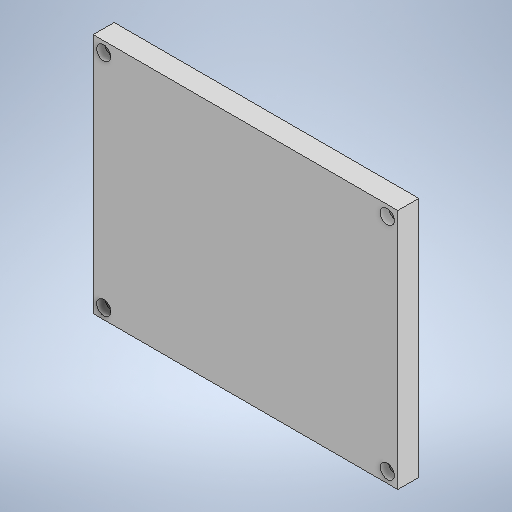
# Autodesk Inventor part: boden
Saved by Autodesk Inventor 2027 (Build 310192060, 192F)
## iProperties
Created: 2026-06-16
Part Number: boden
Material: Generic
Document SubType Name: Modeling
Designer: Felix
Density: 1 g/cm^3
Appearance: Default
Author: Felix
Autodesk Inventor part; units mm, degrees
ref_plane "YZ Plane" through (0, 0, 0) normal (1, 0, 0) x (0, 1, 0)
ref_plane "XZ Plane" through (0, 0, 0) normal (0, 1, 0) x (-1, 0, 0)
ref_plane "XY Plane" through (0, 0, 0) normal (0, 0, 1) x (1, 0, 0)
sketch "Sketch3" plane through (0, 0, 0) normal (0, 0, 1) x (1, 0, 0)
  line L0 (0, 0) -> (145, 0)
  line L1 (145, 0) -> (145, 115)
  line L2 (145, 115) -> (0, 115)
  line L3 (0, 115) -> (0, 0)
  dimension "d24" = 145
  dimension "d25" = 115
  constraints: 8 end point, 2 parallel, 1 horizontal, 1 perpendicular
  measures "d24" distance of L2.end L1.end
  measures "d25" distance of L1.end L0.end
extrude "Extrusion1" add sketch "Sketch3" along normal blind 10
sketch "Sketch1" plane through (0, 0, 0) normal (0, 0, 1) x (1, 0, 0)
  circle A0 centre (15, 43) radius 2
  circle A1 centre (62, 43) radius 2
  circle A2 centre (15, 20) radius 2
  circle A3 centre (20, 95) radius 2
  circle A4 centre (78, 95) radius 2
  circle A5 centre (20, 63) radius 2
  circle A6 centre (97, 56.9) radius 2
  circle A7 centre (133.9, 56.9) radius 2
  circle A8 centre (97, 20) radius 2
  point P0 (0, 0)
  point P1 (3.899, 77.9301)
  dimension "d0" = 4
  dimension "d1" = 4
  dimension "d2" = 4
  dimension "d3" = 23
  dimension "d4" = 47
  dimension "d6" = 4
  dimension "d7" = 4
  dimension "d8" = 4
  dimension "d9" = 32
  dimension "d10" = 58
  dimension "d11" = 5
  dimension "d12" = 20
  dimension "d13" = 4
  dimension "d14" = 4
  dimension "d15" = 4
  dimension "d16" = 36.9
  dimension "d17" = 36.9
  dimension "d18" = 35
  dimension "d28" = 20
  dimension "d29" = 15
  constraints: 9 centre point, 4 horizontal alignment, 3 vertical alignment
  measures "d0" diameter of A0
  measures "d1" diameter of A1
  measures "d2" diameter of A2
  measures "d3" distance of A2.centre A0.centre
  measures "d4" distance of A1.centre A0.centre
  measures "d6" diameter of A3
  measures "d7" diameter of A4
  measures "d8" diameter of A5
  measures "d9" distance of A5.centre A3.centre
  measures "d10" distance of A4.centre A3.centre
  measures "d11" horizontal distance of A0.centre A5.centre
  measures "d12" vertical distance of A0.centre A5.centre
  measures "d13" diameter of A6
  measures "d14" diameter of A7
  measures "d15" diameter of A8
  measures "d16" distance of A8.centre A6.centre
  measures "d17" distance of A7.centre A6.centre
  measures "d18" horizontal distance of A8.centre A1.centre
  measures "d28" vertical distance of point (0, 0) A2.centre
  measures "d29" horizontal distance of point (0, 0) A2.centre
extrude "Extrusion2" cut sketch "Sketch1" along normal blind 5.7
sketch "Sketch4" plane through (0, 0, 10) normal (0, 0, 1) x (1, 0, 0)
  circle A0 centre (5, 5) radius 3.4
  line L0 (0, 115) -> (0, 0) projected
  line L1 (0, 0) -> (145, 0) projected
  line L2 (0, 115) -> (0, 0) projected
  line L3 (0, 57.5) -> (145, 57.5)
  line L4 (145, 0) -> (145, 115) projected
  line L5 (72.5, 0) -> (72.5, 115)
  line L6 (145, 115) -> (0, 115) projected
  circle A1 centre (5, 5) radius 1.75
  circle A2 centre (5, 110) radius 3.4
  circle A3 centre (5, 110) radius 1.75
  circle A4 centre (140, 5) radius 3.4
  circle A5 centre (140, 5) radius 1.75
  circle A6 centre (140, 110) radius 3.4
  circle A7 centre (140, 110) radius 1.75
  dimension "d32" = 6.8
  dimension "d33" = 5
  dimension "d34" = 5
  dimension "d35" = 3.5
  constraints: 8 centre point, 6 symmetric about line, 4 coincident, 4 end point, 4 midpoint, 6 other
  measures "d32" diameter of A0
  measures "d33" distance from line of L0 A0.centre
  measures "d34" distance from line of L1 A0.centre
  measures "d35" diameter of A1
extrude "Extrusion3" cut sketch "Sketch4" against normal through all contours A1 | A3 | A5 | A7
sketch "Sketch6" plane through (0, 0, 10) normal (0, 0, 1) x (1, 0, 0)
  circle A0 centre (5, 110) radius 1.75 projected
  circle A1 centre (5, 110) radius 3.4
  circle A2 centre (5, 5) radius 1.75 projected
  circle A3 centre (5, 5) radius 3.4
  circle A4 centre (140, 110) radius 1.75 projected
  circle A5 centre (140, 110) radius 3.4
  circle A6 centre (140, 5) radius 1.75 projected
  circle A7 centre (140, 5) radius 3.4
  point P0 (0, 0)
  dimension "d39" = 6.8
  dimension "d40" = 6.8
  dimension "d41" = 6.8
  dimension "d42" = 6.8
  constraints: 4 centre point, 4 coincident
  measures "d39" diameter of A1
  measures "d40" diameter of A3
  measures "d41" diameter of A5
  measures "d42" diameter of A7
extrude "Extrusion4" cut sketch "Sketch6" against normal blind 4
body "Solid1"
